RFIDFRIEND_v1 (Autodesk Fusion 360 design; units mm, degrees)
Autodesk Fusion 360 part; units mm, degrees
cylinder "CylinderPrimitive1" add diameter 42 height 5.5 placed x (1, 0, 0) y (0, 0, -1) z (0, 1, 0) at (0, 0, 0) makes body 1
copy_body "CopyPasteBodies1" bodies 1 makes body 2
move_body "Move1" bodies 2 to x (1, 0, 0) y (0, 1, 0) z (0, 0, 1) at (46, 0, 0)
extrude "Extrude1" cut 1 faces at (53.0712, 5.5, 3.0372) along direction (0, -1, 0) blind 4 on bodies 2 bodies 2
cylinder "CylinderPrimitive2" cut diameter 39 height -0.3 placed x (1, 0, 0) y (0, 0, -1) z (0, 1, 0) at (0, 5.5, 0) bodies 1
cylinder "CylinderPrimitive3" cut diameter 8 height -4.7 placed x (1, 0, 0) y (0, 0, -1) z (0, 1, 0) at (0, 5.2, 0) bodies 1
sketch "Sketch5" plane through (0, 5.5, 0) normal (0, 1, 0) x (-1, 0, 0)
  circle A0 centre (0, 0) radius 19.5
  circle A1 centre (0, 0) radius 21
fillet "Fillet1" radius 1 2 edges at (-19.5789, 0, -7.5939) (26.4211, 0, -7.5939) on bodies 1 2
fillet "Fillet2" radius 0.15 1 edges at (-19.5789, 5.5, 7.5939) on bodies 1 2
fillet "Fillet2" radius 0.15 1 edges at (26.4211, 1.5, -7.5939) on bodies 1 2
